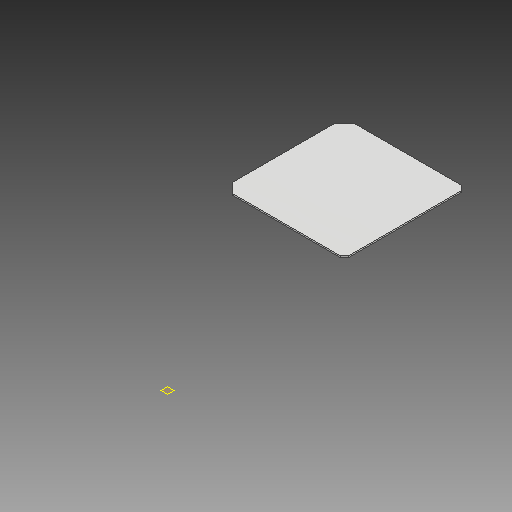
# Autodesk Inventor part: ground plate
Saved by Autodesk Inventor 2018 (Build 220112000, 112)
## iProperties
Part Number: ground plate
Material: Holz
Document SubType Name: Modeling
Designer: Till
Density: 0.570257 g/cm^3
Appearance: Urethan
Author: Till
Autodesk Inventor part; units mm, degrees
ref_plane "YZ Plane" through (0, 0, 0) normal (1, 0, 0) x (0, 1, 0)
ref_plane "XZ Plane" through (0, 0, 0) normal (0, 1, 0) x (-1, 0, 0)
ref_plane "XY Plane" through (0, 0, 0) normal (0, 0, 1) x (1, 0, 0)
ref_plane "Arbeitsebene2" through (86.538, -679.8145, -5.3354) normal (0, 0, 1) x (1, 0, 0)
sketch "Skizze1" plane through (86.538, -679.8145, -5.3354) normal (0, 0, 1) x (1, 0, 0)
  line L0 (-86.538, 679.8145) -> (-486.538, 679.8145) construction
  line L1 (-486.538, 679.8145) -> (-486.538, 1079.8145) construction
  line L2 (-486.538, 1079.8145) -> (-86.538, 1079.8145) construction
  line L3 (-86.538, 1079.8145) -> (-86.538, 679.8145) construction
  line L4 (-458.538, 1083.8145) -> (-490.538, 1051.8145)
  line L5 (-458.538, 1083.8145) -> (-413.2832, 1083.8145) construction
  line L6 (-458.538, 675.8145) -> (-490.538, 707.8145)
  line L7 (-458.538, 675.8145) -> (-413.2832, 675.8145) construction
  line L8 (-82.538, 1069.8145) -> (-96.538, 1083.8145)
  line L9 (-82.538, 1069.8145) -> (-62.739, 1069.8145) construction
  line L10 (-82.538, 689.8145) -> (-96.538, 675.8145)
  line L11 (-82.538, 689.8145) -> (-62.739, 689.8145) construction
  line L12 (-96.538, 1083.8145) -> (-458.538, 1083.8145)
  line L13 (-490.538, 1051.8145) -> (-490.538, 707.8145)
  line L14 (-458.538, 675.8145) -> (-96.538, 675.8145)
  line L15 (-82.538, 689.8145) -> (-82.538, 1069.8145)
  dimension "d0" = 400
  dimension "d1" = 400
  dimension "d4" = 135
  dimension "d5" = 4
  dimension "d6" = 28
  dimension "d7" = 4
  dimension "d8" = 135
  dimension "d9" = 4
  dimension "d10" = 28
  dimension "d11" = 4
  dimension "d12" = 135
  dimension "d13" = 10
  dimension "d14" = 4
  dimension "d15" = 10
  dimension "d16" = 135
  dimension "d17" = 4
  dimension "d18" = 10
  dimension "d19" = 4
  constraints: 32 end point, 5 horizontal, 4 equal length, 2 parallel, 1 perpendicular
  measures "d0" distance of L1.end L2.end
  measures "d1" distance of L0.end L1.end
  measures "d4" angle of L4 L5
  measures "d5" distance from line of L2 L4.start
  measures "d6" distance from line of L1 L4.start
  measures "d7" distance from line of L1 L4.end
  measures "d8" angle of L7 L6
  measures "d9" distance from line of L0 L6.start
  measures "d10" distance from line of L1 L6.start
  measures "d11" distance from line of L1 L6.end
  measures "d12" angle of L9 L8
  measures "d13" distance from line of L2 L8.start
  measures "d14" distance from line of L3 L8.start
  measures "d15" distance from line of L3 L8.end
  measures "d16" angle of L10 L11
  measures "d17" distance from line of L3 L10.start
  measures "d18" distance from line of L0 L10.start
  measures "d19" distance from line of L0 L10.end
extrude "Extrusion1" add sketch "Skizze1" along normal blind 5
